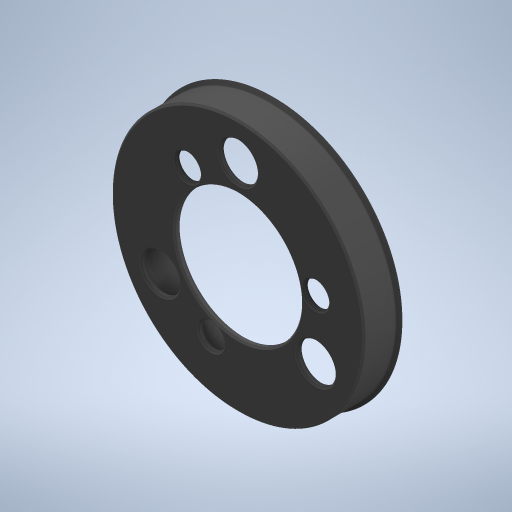
# Autodesk Inventor part: planet_bearing_spacer
Saved by Autodesk Inventor 2023 (Build 270158000, 158)
## iProperties
Created: 2023-11-23
Part Number: planet_bearing_spacer
Material: PC/ABS Plastic
Document SubType Name: Modeling
Designer: aaron
Density: 0.357273 g/cm^3
Appearance: Smooth - White
Author: aaron
Autodesk Inventor part; units mm, degrees
ref_plane "YZ Plane" through (0, 0, 0) normal (1, 0, 0) x (0, 1, 0)
ref_plane "XZ Plane" through (0, 0, 0) normal (0, 1, 0) x (-1, 0, 0)
ref_plane "XY Plane" through (0, 0, 0) normal (0, 0, 1) x (1, 0, 0)
sketch "Sketch1" plane through (0, 0, 0) normal (0, 0, 1) x (1, 0, 0)
  circle A0 centre (0, 0) radius 40.05
  circle A1 centre (0, 0) radius 34.925
  dimension "d0" = 80.1
  dimension "d1" = 69.85
  constraints: 2 centre point, 2 coincident
  measures "d0" diameter of A0
  measures "d1" diameter of A1
extrude "Extrusion1" add sketch "Sketch1" along normal blind 9.6
sketch "Sketch2" plane through (0, 0, 9.6) normal (0, 0, 1) x (1, 0, 0)
  circle A0 centre (0, 0) radius 20
  circle A1 centre (0, 0) radius 40.05 projected
  line L0 (0, 0) -> (0, 61.5181)
  circle A2 centre (0, 0) radius 28.5
  circle A3 centre (0, 0) radius 25
  line L1 (0, 0) -> (-40.7696, 48.5873)
  circle A4 centre (0, 28.5) radius 6
  circle A5 centre (-16.0697, 19.1511) radius 4
  circle A6 centre (-24.6817, -14.25) radius 6
  circle A7 centre (-8.5505, -23.4923) radius 4
  circle A8 centre (24.6817, -14.25) radius 6
  circle A9 centre (24.6202, 4.3412) radius 4
  point P0 (21.1514, -19.1015)
  point P1 (28.352, 2.9011)
  point P2 (23.6127, 8.2122)
  point P3 (19.0171, -16.228)
  point P4 (24.9974, 0.359)
  point P5 (27.6344, 6.9708)
  point P6 (23.5624, -8.3553)
  point P7 (27.1181, -8.7669)
  dimension "d5" = 57
  dimension "d6" = 50
  dimension "d4" = 40
  dimension "d7" = 12
  dimension "d8" = 40
  dimension "d9" = 8
  dimension "d12" = 360
  constraints: 7 centre point, 4 end point, 3 coincident, 2 point on line, 1 vertical, 19 other
  measures "d4" diameter of A0
  measures "d7" diameter of A4
  measures "d8" angle of L1 L0
  measures "d9" diameter of A5
extrude "Extrusion2" add sketch "Sketch2" along normal blind 2 contours A0 L0 A4 A3 A9 A8 A7 A6 A5 L1 | A0 L1 A5 A3 A4 L0 | A3 A5 A2 A4 | A4 A2 A9 A3 | A3 A6 A2 A5 | A2 A5 L1 A1 L0 A4 | A4 L0 A1 L1 A5 A2 A6 A7 A8 A9 | A9 A2 A8 A3 | A3 A7 A2 A6 | A3 A8 A2 A7
sketch "Sketch3" plane through (0, 0, 0) normal (0, 0, -1) x (-1, 0, 0)
  circle A0 centre (0, 0) radius 40.05 projected
  circle A1 centre (0, 0) radius 41.05
  dimension "d16" = 1
  constraints: 1 centre point
  measures "d16" radial gap between concentric circles of A0 A1
extrude "Extrusion3" add sketch "Sketch3" against normal blind 1
chamfer "Chamfer1" distance 0.5 angle 45 2 edges at (-40.05, 0, 1) (41.05, 0, 1)
chamfer "Chamfer2" distance 1 angle 45 1 edges at (-34.925, 0, 0)
chamfer "Chamfer3" distance 0.5 angle 45 1 edges at (41.05, 0, 0)
chamfer "Chamfer4" distance 0.5 angle 45 15 edges at (-40.05, 0, 11.6) (-6, 28.5, 11.6) (-20.0697, 19.1511, 11.6) (18.6817, -14.25, 11.6) (20.6202, 4.3412, 11.6) (-30.6817, -14.25, 11.6) (-12.5505, -23.4923, 11.6) (-20, 0, 11.6) (-20, 0, 9.6) (-12.5505, -23.4923, 9.6) (-30.6817, -14.25, 9.6) (20.6202, 4.3412, 9.6) (18.6817, -14.25, 9.6) (-6, 28.5, 9.6) (-20.0697, 19.1511, 9.6)
body "Solid1"
